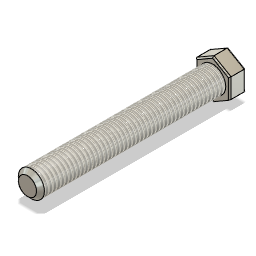
0.163.0723 - Vis H - M10-70_26 (Autodesk Fusion 360 design; units mm, degrees)
Autodesk Fusion 360 part; units mm, degrees
sketch "Sketch1" plane through (0, 0, 0) normal (0, 0, 1) x (1, 0, 0)
  circle A0 centre (0, 0) radius 5
  dimension "d1" = 10
  constraint coincident A0.centre origin
  measures "d1" diameter of A0
extrude "Extrude1" add sketch "Sketch1" along normal blind 70
thread "Thread1" "ISO Metric profile 10.0 M10x1.5 6g" major diameter 9.85 minor diameter 8.141 pitch 1.5 angle 60 resizes the face on face at (4.9752, -0.4978, 46.6667)
sketch "Sketch2" plane through (0, 0, 0) normal (0, 0, -1) x (-1, 0, 0)
  circle A0 centre (0, 0) radius 4.925
  line L0 (4.925, 2.8435) -> (0, 5.6869) construction
  line L1 (0, 5.6869) -> (-4.925, 2.8435) construction
  line L2 (-4.925, 2.8435) -> (-4.925, -2.8435) construction
  line L3 (-4.925, -2.8435) -> (0, -5.6869) construction
  line L4 (0, -5.6869) -> (4.925, -2.8435) construction
  line L5 (4.925, -2.8435) -> (4.925, 2.8435) construction
  line L6 (0, 7.419) -> (-6.425, 3.7095)
  line L7 (-6.425, 3.7095) -> (-6.425, -3.7095)
  line L8 (-6.425, -3.7095) -> (0, -7.419)
  line L9 (0, -7.419) -> (6.425, -3.7095)
  line L10 (6.425, -3.7095) -> (6.425, 3.7095)
  line L11 (6.425, 3.7095) -> (0, 7.419)
  dimension "d4" = 1.5
  constraint coincident A0.centre origin
extrude "Extrude2" add sketch "Sketch2" along normal blind 6 contours A0 | L6 L7 L8 L9 L10 L11
fillet "Fillet1" radius 0.5 11 edges at (3.2125, -5.5642, -6) (-3.2125, -5.5642, -6) (-6.425, 0, -6) (-3.2125, 5.5642, -6) (3.2125, 5.5642, -6) (6.425, 0, -6) (-3.2125, -5.5642, 0) (-6.425, 0, 0) (-3.2125, 5.5642, 0) (3.2125, 5.5642, 0) (6.425, 0, 0)
chamfer "Chamfer1" distance 1.5 angle 45 1 edges at (-4.5917, -1.781, 70)
